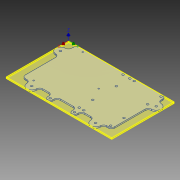
# Autodesk Inventor part: Oberplatte
Saved by Autodesk Inventor 2019.4 (Build 234330000, 330)
## iProperties
Part Number: Oberplatte
Material: Aluminium 6061
Document SubType Name: Modeling
Designer: rYan
Mass: 68.1021 g
Surface Area: 266.585 cm^2
Volume: 25.223 cm^3
Density: 2.7 g/cm^3
Appearance: Aluminium - flach
Author: rYan
Autodesk Inventor part; units mm, degrees
ref_plane "YZ Plane" through (0, 0, 0) normal (1, 0, 0) x (0, 1, 0)
ref_plane "XZ Plane" through (0, 0, 0) normal (0, 1, 0) x (-1, 0, 0)
ref_plane "XY Plane" through (0, 0, 0) normal (0, 0, 1) x (1, 0, 0)
sketch "Skizze1" plane through (0, 0, 0) normal (0, 0, 1) x (1, 0, 0)
  line L0 (-70, 22.5) -> (-75, 22.5)
  line L1 (-75, 7.5) -> (-70, 7.5)
  line L2 (70, 22.5) -> (75, 22.5)
  line L3 (75, 7.5) -> (70, 7.5)
  arc A0 (-75, 22.5) -> (-75, 7.5) centre (-75, 15) ccw
  arc A1 (-57.5, -55) -> (-42.5, -55) centre (-50, -55) ccw
  arc A2 (75, 7.5) -> (75, 22.5) centre (75, 15) ccw
  arc A3 (42.5, -55) -> (57.5, -55) centre (50, -55) ccw
  line L4 (-70, 22.5) -> (-70, 35)
  line L5 (-70, -50) -> (-70, 7.5)
  line L6 (70, 35) -> (70, 22.5)
  line L7 (70, 7.5) -> (70, -50)
  line L8 (0, 54.5) -> (0, -82) projected
  line L9 (-115.5, 0) -> (115.5, 0) projected
  line L10 (-70, 35) -> (70, 35)
  line L11 (23, -50) -> (23, -57)
  line L12 (15, -50) -> (15, -57)
  line L13 (-15, -50) -> (-15, -57)
  line L14 (-23, -50) -> (-23, -57)
  arc A4 (15, -57) -> (23, -57) centre (19, -57) ccw
  arc A5 (-23, -57) -> (-15, -57) centre (-19, -57) ccw
  line L15 (15, -50) -> (-15, -50)
  line L16 (57.5, -50) -> (57.5, -55)
  line L17 (42.5, -55) -> (42.5, -50)
  line L18 (-42.5, -55) -> (-42.5, -50)
  line L19 (-57.5, -55) -> (-57.5, -50)
  line L20 (70, -50) -> (57.5, -50)
  line L21 (42.5, -50) -> (23, -50)
  line L22 (-23, -50) -> (-42.5, -50)
  line L23 (-57.5, -50) -> (-70, -50)
  point P0 (0, 0)
  dimension "d0" = 85
  dimension "d2" = 15
  dimension "d6" = 75
  dimension "d21" = 15
  dimension "d71" = 35
  dimension "d72" = 70
  dimension "d73" = 7
  dimension "d74" = 38
  dimension "d75" = 8
  dimension "d90" = 15
  dimension "d91" = 55
  dimension "d92" = 50
  constraints: 44 end point, 12 point on circle, 12 tangent, 11 parallel, 10 perpendicular, 6 centre point, 5 collinear, 4 vertical, 3 horizontal, 9 other
  measures "d0" distance of L6.start L7.end
  measures "d2" distance between parallel lines of L0 L1
  measures "d6" distance from line of L8 A0.centre
  measures "d21" distance from line of L9 A0.centre
  measures "d71" distance between parallel lines of L10 L9
  measures "d72" distance between parallel lines of L5 L8
  measures "d73" distance from line of A4.centre L15
  measures "d74" distance of A5.centre A4.centre
  measures "d75" distance between parallel lines of L14 L13
  measures "d90" distance between parallel lines of L16 L17
  measures "d91" distance from line of L9 A3.centre
  measures "d92" distance from line of L8 A3.centre
extrude "Extrusion1" add sketch "Skizze1" along normal blind 2
sketch "Skizze2" plane through (0, 0, 2) normal (0, 0, 1) x (1, 0, 0)
  arc A0 (-75, 22.5) -> (-75, 7.5) centre (-75, 15) ccw projected
  arc A1 (-57.5, -55) -> (-42.5, -55) centre (-50, -55) ccw projected
  arc A2 (75, 7.5) -> (75, 22.5) centre (75, 15) ccw projected
  arc A3 (42.5, -55) -> (57.5, -55) centre (50, -55) ccw projected
  point P0 (0, 0)
  constraints: 4 coincident
hole "Montage" at (-75, 15, 2) at (75, 15, 2) at (50, -55, 2) at (-50, -55, 2) direction (0, 0, -1) diameter 3.2 end through all
fillet "Rundung1" radius 5 16 edges at (-70, 7.5, 1) (-70, 35, 1) (-70, -50, 1) (-70, 22.5, 1) (70, 35, 1) (70, 22.5, 1) (70, 7.5, 1) (70, -50, 1) (23, -50, 1) (15, -50, 1) (-15, -50, 1) (-23, -50, 1) (57.5, -50, 1) (42.5, -50, 1) (-57.5, -50, 1) (-42.5, -50, 1)
sketch "Skizze3" plane through (0, 0, 2) normal (0, 0, 1) x (1, 0, 0)
  line L0 (0, 54.5) -> (0, -82) projected
  line L1 (-115.5, 0) -> (115.5, 0) projected
  line L2 (65.5, -26) -> (16.5, -26) construction
  line L3 (16.5, -26) -> (16.5, 32) construction
  line L4 (16.5, 32) -> (65.5, 32) construction
  line L5 (65.5, 32) -> (65.5, -26) construction
  line L6 (16.5, -47) -> (65.5, -47) construction
  line L7 (65.5, -47) -> (65.5, 11) construction
  line L8 (65.5, 11) -> (16.5, 11) construction
  line L9 (16.5, 11) -> (16.5, -47) construction
  point P0 (0, 0)
  dimension "d23" = 49
  dimension "d24" = 58
  dimension "d25" = 32
  dimension "d26" = 16.5
  dimension "d94" = 49
  dimension "d95" = 58
  dimension "d97" = 47
  constraints: 16 end point, 8 coincident, 4 parallel, 2 horizontal, 2 perpendicular, 1 collinear
  measures "d23" distance of L3.end L4.end
  measures "d24" distance of L2.end L3.end
  measures "d25" distance between parallel lines of L1 L4
  measures "d26" distance between parallel lines of L0 L3
  measures "d94" distance of L8.end L7.end
  measures "d95" distance of L7.end L6.end
  measures "d97" distance between parallel lines of L6 L1
hole "RPi" at (65.5, -26, 2) at (16.5, -26, 2) at (65.5, 32, 2) at (16.5, 32, 2) at (16.5, 11, 2) at (65.5, 11, 2) at (65.5, -47, 2) at (16.5, -47, 2) direction (0, 0, -1) diameter 3.2 end through all
sketch "Skizze4" plane through (0, 0, 2) normal (0, 0, 1) x (1, 0, 0)
  circle A0 centre (65.5, 32) radius 1.6 projected
  line L0 (65.5, 32) -> (23.5, 32) construction
  line L1 (23.5, 32) -> (23.5, -47) construction
  line L2 (23.5, -47) -> (65.5, -47) construction
  line L3 (65.5, -47) -> (65.5, 32) construction
  point P0 (0, 0)
  dimension "d34" = 42
  dimension "d35" = 79
  constraints: 8 end point, 3 coincident, 2 parallel, 1 horizontal, 1 perpendicular
  measures "d34" distance of L2.end L1.end
  measures "d35" distance of L1.end L0.end
hole "Jetson" at (65.5, -47, 2) at (23.5, -47, 2) at (23.5, 32, 2) direction (0, 0, -1) diameter 3.2 end through all
sketch "Skizze6" plane through (0, 0, 2) normal (0, 0, 1) x (1, 0, 0)
  line L0 (0, 54.5) -> (0, -82) projected
  line L1 (-115.5, 0) -> (115.5, 0) projected
  line L2 (62.5, -50) -> (65, -50) construction
  line L3 (65, 35) -> (-65, 35) construction
  arc A0 (15, -57) -> (23, -57) centre (19, -57) ccw projected
  arc A1 (-23, -57) -> (-15, -57) centre (-19, -57) ccw projected
  point P0 (0, 0)
  point P1 (6, 32)
  point P2 (-65, -50)
  point P3 (23, -50)
  point P4 (28, -50)
  point P5 (57.5, -50)
  dimension "d61" = 3
  dimension "d63" = 6
  constraints: 2 coincident
  measures "d61" distance from line of point (6, 32) L3
  measures "d63" distance from line of L0 point (6, 32)
hole "Kameras oben" at (19, -57, 2) at (6, 32, 2) at (-19, -57, 2) direction (0, 0, -1) diameter 3.2 end through all
sketch "Skizze7" plane through (0, 0, 2) normal (0, 0, 1) x (1, 0, 0)
  line L0 (0, 54.5) -> (0, -82) projected
  line L1 (-115.5, 0) -> (115.5, 0) projected
  point P0 (0, 0)
  point P1 (-56, 31)
  point P2 (-56, -46)
  point P3 (6, -6)
  dimension "d76" = 56
  dimension "d78" = 56
  dimension "d79" = 46
  dimension "d81" = 31
  dimension "d89" = 6
  dimension "d93" = 6
  measures "d76" distance from line of L0 point (-56, 31)
  measures "d78" distance from line of point (-56, -46) L0
  measures "d79" distance from line of point (-56, -46) L1
  measures "d81" distance from line of point (-56, 31) L1
  measures "d89" distance from line of point (6, -6) L0
  measures "d93" distance from line of point (6, -6) L1
hole "Mainboard" at (-56, 31, 2) at (-56, -46, 2) at (6, -6, 2) direction (0, 0, -1) diameter 2.1 end through all
